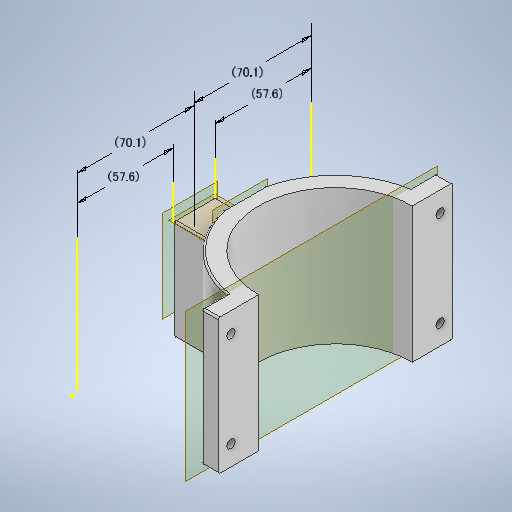
# Autodesk Inventor part: motor_mount
Saved by Autodesk Inventor 2025.2 (Build 292293000, 293)
## iProperties
Created: 2024-12-14
Part Number: motor_mount
Material: 一般
Document SubType Name: Modeling
Designer: mahhy
Density: 1 g/cm^3
Appearance: 既定
Author: mahhy
## iProperties of the stored document motor_mount1_3D プリント.ipt
Created: 2024-12-17
Part Number: motor_mount1_3D プリント
Material: 一般
Document SubType Name: Modeling
Designer: mahhy
Density: 1 g/cm^3
Appearance: 既定
Author: mahhy
Autodesk Inventor part; units mm, degrees
ref_plane "YZ Plane" through (0, 0, 0) normal (1, 0, 0) x (0, 1, 0)
ref_plane "XZ Plane" through (0, 0, 0) normal (0, 1, 0) x (-1, 0, 0)
ref_plane "XY Plane" through (0, 0, 0) normal (0, 0, 1) x (1, 0, 0)
sketch "スケッチ1" plane through (0, 0, 0) normal (0, 1, 0) x (-1, 0, 0)
  line L0 (0, 0) -> (70, 0)
  line L1 (70, 0) -> (70, -170)
  line L2 (70, -170) -> (0, -170)
  line L3 (0, -170) -> (0, 0)
  arc A0 (0, -118.9591) -> (0, -26.9591) centre (0, -72.9591) ccw
  arc A1 (0, -128.9591) -> (0, -16.9591) centre (0, -72.9591) ccw
  line L4 (10, -17.8592) -> (0, -17.8592)
  line L5 (0, -17.8592) -> (0, -2.8592)
  line L6 (0, -2.8592) -> (10, -2.8592)
  line L7 (10, -2.8592) -> (10, -17.8592)
  line L8 (10, -128.0591) -> (0, -128.0591)
  line L9 (0, -128.0591) -> (0, -143.0591)
  line L10 (0, -143.0591) -> (10, -143.0591)
  line L11 (10, -143.0591) -> (10, -128.0591)
  line L12 (54.5871, -60.4591) -> (54.5871, -85.4591)
  point P0 (54.5871, -72.9591)
  point P1 (46, -72.9591)
  dimension "d8" = 70
  dimension "d9" = 170
  dimension "d10" = 46
  dimension "d11" = 56
  dimension "d12" = 10
  dimension "d13" = 10
  dimension "d14" = 15
  dimension "d15" = 15
  dimension "d17" = 25
  constraints: 24 end point, 9 point on circle, 5 parallel, 3 horizontal, 3 perpendicular, 2 centre point, 2 vertical, 1 coincident, 1 midpoint, 10 other
  measures "d8" distance of L1.end L2.end
  measures "d9" distance of L0.end L1.end
  measures "d10" radius of A0
  measures "d11" radius of A1
  measures "d14" distance of L6.end L4.start
  measures "d15" distance of L10.end L8.start
  measures "d17" distance of L12.start L12.end
extrude "押し出し1" add sketch "スケッチ1" along normal blind 81 contours L6 L7 A1 L3 | A1 L4 L3 | L4 A1 L12 L8 L3 A0 | L3 A1 L11 L10 | L3 L8 A1
ref_plane "作業平面1" through (-54.5871, 0, -85.4591) normal (-1, 0, 0) x (0, 0, 1)
sketch "スケッチ2" plane through (-54.5871, 0, -85.4591) normal (-1, 0, 0) x (0, 0, 1)
  line L0 (-33.5, 81) -> (58.5, 81) projected
  line L1 (0, 60.4) -> (25, 60.4)
  line L2 (25, 60.4) -> (25, 0)
  line L3 (25, 0) -> (0, 0)
  line L4 (0, 0) -> (0, 60.4)
  line L5 (0, 81) -> (25, 81) projected
  line L6 (0, 0) -> (0, 81) projected
  line L7 (0, 0) -> (25, 0) projected
  line L8 (-57.5999, 0) -> (-57.5999, 81) projected
  line L9 (82.5999, 0) -> (82.5999, 81) projected
  line L10 (-57.5999, 81) -> (82.5999, 0)
  line L11 (-57.5999, 0) -> (-42.5999, 0) projected
  line L12 (-57.5999, 0) -> (82.5999, 81)
  line L13 (12.5, 40.5) -> (12.5, 0) construction
  point P0 (85.4591, 0)
  point P1 (12.5, 81)
  point P2 (12.5, 81)
  point P3 (0, 40.5)
  dimension "d21" = 25
  dimension "d22" = 60.4
  dimension "d50" = 20.6
  dimension "d92" = 40.5
  dimension "d93" = 40.5
  dimension "d96" = 12.5
  constraints: 14 end point, 5 midpoint, 2 parallel, 1 horizontal, 1 perpendicular, 1 point on line
  measures "d21" distance of L2.end L3.end
  measures "d22" distance of L1.end L2.end
  measures "d50" distance between parallel lines of L0 L1
  measures "d92" distance from line of L0 point (0, 40.5)
  measures "d93" distance from line of L3 point (0, 40.5)
  measures "d96" distance between parallel lines of L2 L13
extrude "押し出し2" add sketch "スケッチ2" along normal blind 30 contours L1 L2 L12 L10 L4 | L10 L12 L4 | L2 L10 L12 | L12 L10 L2 L3 L4
ref_plane "作業平面3" through (-84.5871, 0, -85.4591) normal (-1, 0, 0) x (0, 0, 1)
sketch "スケッチ4" plane through (-84.5871, 0, -85.4591) normal (-1, 0, 0) x (0, 0, 1)
  line L0 (2.45, 50.4) -> (22.55, 50.4)
  line L1 (22.55, 50.4) -> (22.55, 10.4)
  line L2 (22.55, 10.4) -> (2.45, 10.4)
  line L3 (2.45, 10.4) -> (2.45, 50.4)
  line L4 (0, 60.4) -> (25, 60.4) projected
  line L5 (0, 0) -> (0, 60.4) projected
  line L6 (0, 60.4) -> (0, 0) projected
  line L7 (0, 0) -> (25, 0) projected
  line L8 (7.6, 54.5) -> (17.3, 54.5)
  line L9 (7.7, 6.3) -> (17.4, 6.3)
  line L10 (25, 60.4) -> (0, 60.4) projected
  line L11 (0, 81) -> (25, 81) projected
  line L12 (25, 0) -> (25, 60.4) projected
  point P0 (85.4591, 0)
  point P1 (12.5, 50.4)
  point P2 (12.5, 60.4)
  point P3 (2.45, 30.4)
  point P4 (0, 30.2)
  point P5 (0, 0.35)
  point P6 (25, 60)
  point P7 (12.55, 6.3)
  point P8 (12.45, 54.5)
  point P9 (12.5, 60.4)
  point P10 (12.5, 10.4)
  point P11 (12.55, 40.5)
  point P12 (12.5, 81)
  dimension "d28" = 20.1
  dimension "d29" = 40
  dimension "d52" = 10.4
  dimension "d53" = 2.45
  dimension "d54" = 4.1
  dimension "d55" = 4.1
  dimension "d56" = 4.1
  dimension "d57" = 4.1
  dimension "d58" = 9.7
  dimension "d59" = 9.7
  dimension "d100" = 40.5
  dimension "d101" = 9.9
  dimension "d102" = 40.5
  dimension "d107" = 2.45
  constraints: 12 end point, 7 midpoint, 2 parallel, 1 horizontal, 1 perpendicular, 5 other
  measures "d28" distance of L1.end L2.end
  measures "d29" distance of L0.end L1.end
  measures "d52" distance of the line from the sketch origin of L2
  measures "d53" distance between parallel lines of L5 L3
  measures "d54" distance from line of L0 L8.start
  measures "d55" distance from line of L0 L8.end
  measures "d56" distance from line of L2 L9.start
  measures "d57" distance from line of L2 L9.end
  measures "d58" distance of L8.end L8.start
  measures "d59" distance of L9.end L9.start
  measures "d101" distance from line of L0 point (12.55, 40.5)
  measures "d102" distance of point (12.5, 81) point (12.55, 40.5)
  measures "d107" distance between parallel lines of L12 L1
extrude "押し出し3" cut sketch "スケッチ4" against normal blind 27.5 contours L0 L1 L2 L3
ref_plane "作業平面4" through (-10, 0, -143.0591) normal (-1, 0, 0) x (0, 0, 1)
sketch "スケッチ5" plane through (-10, 0, -143.0591) normal (-1, 0, 0) x (0, 0, 1)
  line L0 (0, 81) -> (15, 81) projected
  line L1 (0, 0) -> (15, 0) projected
  line L2 (125.1998, 81) -> (140.1998, 81) projected
  line L3 (125.1998, 0) -> (140.1998, 0) projected
  point P0 (143.0591, 0)
  point P1 (7.5, 69)
  point P2 (7.5, 12)
  point P3 (132.6998, 69)
  point P4 (132.6998, 12)
  point P5 (7.5, 81)
  point P6 (7.5, 0)
  point P7 (132.6998, 81)
  point P8 (132.6998, 0)
  dimension "d35" = 0
  dimension "d36" = 0
  dimension "d37" = 0
  dimension "d38" = 0
  dimension "d39" = 12
  dimension "d40" = 12
  dimension "d41" = 12
  dimension "d42" = 12
  constraints: 4 midpoint
  measures "d35" horizontal distance of point (7.5, 69) point (7.5, 81)
  measures "d36" horizontal distance of point (7.5, 12) point (7.5, 0)
  measures "d37" horizontal distance of point (132.7, 81) point (132.7, 69)
  measures "d38" horizontal distance of point (132.7, 0) point (132.7, 12)
  measures "d39" distance from line of L0 point (7.5, 69)
  measures "d40" distance from line of L1 point (7.5, 12)
  measures "d41" distance from line of L2 point (132.7, 69)
  measures "d42" distance from line of L3 point (132.7, 12)
hole "穴1" at (-10, 69, -135.5591) at (-10, 12, -135.5591) at (-10, 69, -10.3592) at (-10, 12, -10.3592) direction (1, 0, 0) diameter 5 end through all
sketch "スケッチ6" plane through (-84.5871, 0, -85.4591) normal (-1, 0, 0) x (0, 0, 1)
  line L0 (7.7, 6.3) -> (17.4, 6.3)
  line L1 (7.7, 54.5) -> (17.4, 54.5)
  line L2 (22.55, 10.4) -> (2.45, 10.4) projected
  line L3 (2.45, 50.4) -> (22.55, 50.4) projected
  point P0 (85.4591, 0)
  point P1 (12.55, 6.3)
  point P2 (12.55, 54.5)
  point P3 (12.5, 10.4)
  point P4 (12.5, 50.4)
  dimension "d63" = 9.7
  dimension "d64" = 9.7
  dimension "d65" = 4.1
  dimension "d66" = 4.1
  constraints: 4 end point, 4 midpoint, 2 horizontal
  measures "d63" distance of L0.start L0.end
  measures "d64" distance of L1.start L1.end
  measures "d65" distance between parallel lines of L2 L0
  measures "d66" distance between parallel lines of L3 L1
hole "穴2" at (-84.5871, 54.5, -77.7591) at (-84.5871, 54.5, -68.0591) at (-84.5871, 6.3, -77.7591) at (-84.5871, 6.3, -68.0591) direction (1, 0, 0) diameter 4 depth 10
ref_plane "作業平面5" through (-84.5871, 60.4, -85.4591) normal (0, 1, 0) x (1, 0, 0)
sketch "スケッチ8" plane through (-84.5871, 60.4, -85.4591) normal (0, 1, 0) x (1, 0, 0)
  line L0 (14.2, -17.5) -> (21.2, -17.5)
  line L1 (21.2, -17.5) -> (21.2, -7.5)
  line L2 (21.2, -7.5) -> (14.2, -7.5)
  line L3 (14.2, -7.5) -> (14.2, -17.5)
  line L4 (0, -114.071) -> (0, 86.2117) projected
  line L5 (30, 0) -> (30, -25) projected
  point P0 (84.5871, -85.4591)
  point P1 (14.2, -12.5)
  point P2 (30, -12.5)
  dimension "d87" = 7
  dimension "d88" = 10
  dimension "d89" = 14.2
  constraints: 8 end point, 2 midpoint, 2 parallel, 1 horizontal, 1 perpendicular
  measures "d87" distance of L2.end L1.end
  measures "d88" distance of L1.end L0.end
  measures "d89" distance from line of L4 point (14.2, -12.5)
extrude "押し出し5" cut sketch "スケッチ8" against normal blind 12
fillet "フィレット2" radius 1 23 edges at (-10, 40.5, -143.0591) (-10, 81, -135.5591) (-5, 81, -143.0591) (-5, 0, -143.0591) (-10, 0, -135.5591) (-10, 0, -10.3592) (-5, 0, -2.8592) (-69.5871, 0, -85.4591) (-69.5871, 0, -60.4591) (-84.5871, 0, -72.9591) (-84.5871, 30.2, -85.4591) (-69.5871, 60.4, -85.4591) (-84.5871, 60.4, -72.9591) (-84.5871, 30.2, -60.4591) (-69.5871, 60.4, -60.4591) (-38.6854, 0, -32.4692) (-38.6854, 0, -113.4491) (-10, 40.5, -2.8592) (-5, 81, -2.8592) (-10, 81, -10.3592) (-38.6854, 81, -32.4692) (-38.6854, 81, -113.4491) (-54.5871, 81, -72.9591)
sketch "スケッチ9" plane through (-84.5871, 0, -85.4591) normal (-1, 0, 0) x (0, 0, 1)
  line L0 (2.45, 50.4) -> (22.55, 50.4) projected
  line L1 (2.45, 50.4) -> (22.55, 50.4) projected
  line L2 (-57.5999, 80) -> (-57.5999, 1) projected
  line L3 (82.5999, 1) -> (82.5999, 80) projected
  line L4 (0, 59.4) -> (0, 80) projected
  line L5 (25, 59.4) -> (25, 80) projected
  point P0 (85.4591, 0)
  point P1 (12.5, 50.4)
  point P2 (12.5, 50.4)
  point P3 (12.5, 50.4)
  dimension "d103" = 70.0999
  dimension "d104" = 70.0999
  dimension "d105" = 57.5999
  dimension "d106" = 57.5999
  constraints: 3 midpoint
  measures "d103" distance from line of point (12.5, 50.4) L2
  measures "d104" distance from line of L3 point (12.5, 50.4)
  measures "d105" distance between parallel lines of L2 L4
  measures "d106" distance between parallel lines of L3 L5
